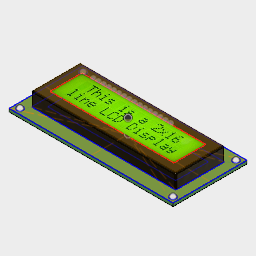
BaseStationCase (Autodesk Fusion 360 archive; units mm, degrees)
design "1602 LCD"
Autodesk Fusion 360 part; units mm, degrees
sketch "Sketch1" plane through (0, 0, 0) normal (0, 1, 0) x (1, 0, 0)
  line L0 (40.35, -18.2) -> (-40.35, -18.2)
  line L1 (-40.35, -18.2) -> (-40.35, 18.2)
  line L2 (-40.35, 18.2) -> (40.35, 18.2)
  line L3 (40.35, 18.2) -> (40.35, -18.2)
  line L4 (40.35, -18.2) -> (-40.35, 18.2) construction
  line L5 (-40.35, -18.2) -> (40.35, 18.2) construction
  line L6 (35.5, -12) -> (-35.5, -12)
  line L7 (-35.5, -12) -> (-35.5, 12)
  line L8 (-35.5, 12) -> (35.5, 12)
  line L9 (35.5, 12) -> (35.5, -12)
  line L10 (35.5, -12) -> (-35.5, 12) construction
  line L11 (-35.5, -12) -> (35.5, 12) construction
  line L12 (0, 18.2) -> (0, -18.2) construction
  line L13 (-40.35, 0) -> (40.35, 0) construction
  circle A0 centre (37.675, 15.525) radius 1.575
  circle A1 centre (-37.675, -15.525) radius 1.575
  circle A2 centre (37.675, -15.525) radius 1.575
  circle A3 centre (-32.35, 15.2) radius 0.5
  circle A4 centre (-37.675, 15.525) radius 1.575
  circle A5 centre (-29.81, 15.2) radius 0.5
  circle A6 centre (-27.27, 15.2) radius 0.5
  circle A7 centre (-24.73, 15.2) radius 0.5
  circle A8 centre (-22.19, 15.2) radius 0.5
  circle A9 centre (-19.65, 15.2) radius 0.5
  circle A10 centre (-17.11, 15.2) radius 0.5
  circle A11 centre (-14.57, 15.2) radius 0.5
  circle A12 centre (-12.03, 15.2) radius 0.5
  circle A13 centre (-9.49, 15.2) radius 0.5
  circle A14 centre (-6.95, 15.2) radius 0.5
  circle A15 centre (-4.41, 15.2) radius 0.5
  circle A16 centre (-1.87, 15.2) radius 0.5
  circle A17 centre (0.67, 15.2) radius 0.5
  circle A18 centre (3.21, 15.2) radius 0.5
  circle A19 centre (5.75, 15.2) radius 0.5
  line L14 (31.5, -8) -> (-31.5, -8)
  line L15 (-31.5, -8) -> (-31.5, 8)
  line L16 (-31.5, 8) -> (31.5, 8)
  line L17 (31.5, 8) -> (31.5, -8)
  dimension "d1" = 80.7
  dimension "d2" = 36.4
  dimension "d3" = 71
  dimension "d4" = 24
  dimension "d52" = 1
  dimension "d53" = 8
  dimension "d54" = 3
  dimension "d57" = 2.54
  dimension "d58" = 0
  dimension "d59" = 4
  dimension "d64" = 3.15
  dimension "d65" = 2.675
  dimension "d66" = 2.675
  constraint perpendicular L0 L1
  constraint parallel L0 L2
  constraint parallel L1 L3
  constraint horizontal L0
  constraint coincident L4 origin
  constraint coincident L5 origin
  constraint perpendicular L6 L7
  constraint parallel L6 L8
  constraint parallel L7 L9
  constraint horizontal L6
  constraint coincident L10 origin
  constraint coincident L11 origin
  constraint midpoint L2 origin
  constraint midpoint L0 origin
  constraint midpoint L1 origin
  constraint midpoint L3
  measures "d52" diameter of A3
  measures "d64" diameter of A4
extrude "Extrude1" add sketch "Sketch1" against normal blind 1.6 contours L0 L1 L2 L3 | L6 L7 L8 L9 | L14 L15 L16 L17
extrude "Extrude2" add sketch "Sketch1" along normal blind 7 contours L6 L7 L8 L9 | L14 L15 L16 L17
fillet "Fillet2" radius 0.5 8 edges at (-35.5, 3.5, -12) (-35.5, 3.5, 12) (35.5, 3.5, 12) (35.5, 3.5, -12) (35.5, 7, 0) (0, 7, -12) (-35.5, 7, 0) (0, 7, 12)
sketch "Sketch6" plane through (0, 7, 0) normal (0, 1, 0) x (-1, 0, 0)
  line L0 (35, 11.5) -> (-35, 11.5)
  line L1 (-35, 11.5) -> (-35, -11.5)
  line L2 (-35, -11.5) -> (35, -11.5)
  line L3 (35, -11.5) -> (35, 11.5)
equation "d65 = d64 / 2 + 1.1 mm"
equation "d66 = d65"
